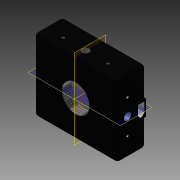
# Autodesk Inventor part: dragonfly2Camera
Saved by Autodesk Inventor 2013 (Build 170138000, 138)
## iProperties
Created: 2014-07-04
Part Number: dragonfly2Camera
Material: Aluminum 6061
Document SubType Name: Modeling
Designer: Nano
Density: 2.71 g/cm^3
Mass: 338.154 g
Surface Area: 170.988 cm^2
Volume: 124.78 cm^3
Author: Nano
Autodesk Inventor part; units mm, degrees
ref_plane "YZ Plane" through (0, 0, 0) normal (1, 0, 0) x (0, 1, 0)
ref_plane "XZ Plane" through (0, 0, 0) normal (0, 1, 0) x (-1, 0, 0)
ref_plane "XY Plane" through (0, 0, 0) normal (0, 0, 1) x (1, 0, 0)
sketch "Sketch1" plane through (0, 0, 0) normal (0, 1, 0) x (-1, 0, 0)
  line L0 (-37.465, -32.512) -> (37.465, -32.512)
  line L1 (37.465, -32.512) -> (37.465, 32.512)
  line L2 (37.465, 32.512) -> (-37.465, 32.512)
  line L3 (-37.465, 32.512) -> (-37.465, -32.512)
  line L4 (-37.465, -32.512) -> (37.465, 32.512) construction
  line L5 (37.465, -32.512) -> (-37.465, 32.512) construction
  point P0 (0, 0)
  point P1 (0, 0)
  dimension "d0" = 74.93
  dimension "d1" = 65.024
  constraints: 12 end point, 2 midpoint, 2 parallel, 1 horizontal, 1 perpendicular
  measures "d0" distance of L2.end L1.end
  measures "d1" distance of L1.end L0.end
extrude "Extrusion1" add sketch "Sketch1" along normal blind 25.654
sketch "Sketch2" plane through (-37.465, 0, 32.512) normal (0, 0, 1) x (1, 0, 0)
  line L0 (74.93, 0) -> (74.93, 25.654) projected
  line L1 (0, 25.654) -> (74.93, 25.654) projected
  line L2 (0, 0) -> (0, 25.654) projected
  circle A0 centre (37.465, 16.764) radius 3.175
  point P0 (37.465, 0)
  dimension "d4" = 6.35
  dimension "d5" = 37.465
  dimension "d6" = 37.465
  dimension "d7" = 8.89
  constraints: 1 centre point
  measures "d4" diameter of A0
  measures "d5" distance from line of L0 A0.centre
  measures "d6" distance from line of L2 A0.centre
  measures "d7" distance from line of L1 A0.centre
extrude "Extrusion2" cut sketch "Sketch2" against normal blind 5.588
sketch "Sketch3" plane through (-37.465, 0, 32.512) normal (0, 0, 1) x (1, 0, 0)
  circle A0 centre (37.465, 16.764) radius 3.175 projected
  line L0 (74.93, 0) -> (74.93, 25.654) projected
  line L1 (0, 0) -> (0, 25.654) projected
  circle A1 centre (57.531, 16.764) radius 1.143
  line L2 (37.465, 25.654) -> (37.465, 0) construction
  circle A2 centre (17.399, 16.764) radius 1.143
  dimension "d10" = 2.286
  dimension "d11" = 20.066
  dimension "d12" = 20.066
  dimension "d13" = 37.465
  dimension "d14" = 37.465
  constraints: 2 centre point, 2 end point, 1 symmetric about line, 1 other
  measures "d10" diameter of A1
  measures "d11" distance of A1.centre A0.centre
  measures "d12" distance of A2.centre A0.centre
  measures "d13" distance between parallel lines of L0 L2
  measures "d14" distance between parallel lines of L1 L2
extrude "Extrusion3" cut sketch "Sketch3" against normal blind 4.318 contours A1 | A2
ref_plane "Work Plane1" through (-37.465, 0, 0) normal (0, 0, 1) x (1, 0, 0)
mirror "Mirror1" about plane through (-37.465, 0, 0) normal (0, 0, 1) of "Extrusion2", "Extrusion3"
ref_plane "Work Plane2" through (0, 0, 32.512) normal (1, 0, 0) x (0, 0, -1)
sketch "Sketch4" plane through (37.465, 0, 32.512) normal (1, 0, 0) x (0, 0, -1)
  line L0 (0, 25.654) -> (65.024, 25.654) projected
  circle A0 centre (32.512, 16.6624) radius 3.175
  circle A1 centre (47.6004, 16.6624) radius 1.016
  line L1 (32.512, 25.654) -> (32.512, 0) construction
  circle A2 centre (17.4236, 16.6624) radius 1.016
  dimension "d19" = 6.35
  dimension "d20" = 8.9916
  dimension "d21" = 2.032
  constraints: 3 centre point, 2 end point, 1 symmetric about line, 1 other
  measures "d19" diameter of A0
  measures "d20" distance from line of A0.centre L0
  measures "d21" diameter of A1
extrude "Extrusion4" cut sketch "Sketch4" against normal blind 4.318
mirror "Mirror2" about plane through (0, 0, 32.512) normal (1, 0, 0) of "Extrusion4"
sketch "Sketch5" plane through (0, 25.654, 0) normal (0, 1, 0) x (1, 0, 0)
  circle A0 centre (0, 0) radius 12.319
  dimension "d24" = 24.638
  constraints: 1 centre point
  measures "d24" diameter of A0
extrude "Extrusion5" cut sketch "Sketch5" against normal blind 8.636
sketch "Sketch6" plane through (37.465, 0, 32.512) normal (1, 0, 0) x (0, 0, -1)
  line L0 (0, 25.654) -> (65.024, 25.654) projected
  line L1 (25.2146, 11.43) -> (39.4386, 11.43)
  line L2 (39.4386, 11.43) -> (39.4386, 1.27)
  line L3 (39.4386, 1.27) -> (25.2146, 1.27)
  line L4 (25.2146, 1.27) -> (25.2146, 11.43)
  point P0 (32.512, 0)
  dimension "d27" = 14.224
  dimension "d28" = 10.16
  dimension "d29" = 14.224
  constraints: 8 end point, 2 parallel, 1 horizontal, 1 perpendicular
  measures "d27" distance of L2.end L3.end
  measures "d28" distance of L1.end L2.end
  measures "d29" distance between parallel lines of L0 L1
extrude "Extrusion6" add sketch "Sketch6" along normal blind 1.016
sketch "Sketch7" plane through (38.481, 0, 32.512) normal (1, 0, 0) x (0, 0, -1)
  line L0 (25.2146, 11.43) -> (25.2146, 1.27) projected
  line L1 (39.4386, 1.27) -> (39.4386, 11.43) projected
  line L2 (26.8656, 8.4177) -> (37.7876, 8.4177)
  line L3 (37.7876, 8.4177) -> (37.7876, 2.5757)
  line L4 (37.7876, 2.5757) -> (26.8656, 2.5757)
  line L5 (26.8656, 4.6339) -> (26.8656, 6.3596)
  line L6 (26.8656, 4.6339) -> (29.2737, 2.5757)
  line L7 (26.8656, 5.4967) -> (37.7876, 5.4967) construction
  line L8 (26.8656, 6.3596) -> (29.2737, 8.4177)
  point P0 (32.512, 0)
  dimension "d32" = 5.842
  dimension "d34" = 10.922
  dimension "d35" = 1.651
  dimension "d36" = 1.651
  constraints: 14 end point, 2 parallel, 2 point on line, 2 symmetric about line, 1 horizontal, 1 perpendicular
  measures "d32" distance of L2.end L3.end
  measures "d34" distance of L2.start L2.end
  measures "d35" distance between parallel lines of L0 L5
  measures "d36" distance between parallel lines of L1 L3
extrude "Extrusion7" cut sketch "Sketch7" against normal blind 7.62
fillet "Fillet1" radius 3.175 12 edges at (0, 25.654, -32.512) (37.465, 12.827, -32.512) (37.465, 25.654, 0) (-37.465, 25.654, 0) (-37.465, 12.827, -32.512) (0, 0, -32.512) (37.465, 0, 0) (-37.465, 0, 0) (0, 0, 32.512) (37.465, 12.827, 32.512) (0, 25.654, 32.512) (-37.465, 12.827, 32.512)
equation "\"d5\" = d6"
equation "\"d12\" = d11"
equation "\"d13\" = d14"
equation "\"d35\" = d36"
body "Solid1"
